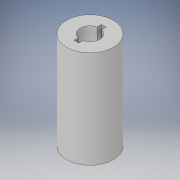
# Autodesk Inventor part: BlenderRoll
Saved by Autodesk Inventor 2019 (Build 230136000, 136)
## iProperties
Created: 2018-06-05
Part Number: BlenderRoll
Material: Ogólny
Document SubType Name: Modeling
Designer: Kamil
Density: 1 g/cm^3
Appearance: Domyślna
Author: Kamil
Autodesk Inventor part; units mm, degrees
ref_plane "YZ Plane" through (0, 0, 0) normal (1, 0, 0) x (0, 1, 0)
ref_plane "XZ Plane" through (0, 0, 0) normal (0, 1, 0) x (-1, 0, 0)
ref_plane "XY Plane" through (0, 0, 0) normal (0, 0, 1) x (1, 0, 0)
sketch "Szkic1" plane through (0, 0, 0) normal (0, 1, 0) x (-1, 0, 0)
  circle A0 centre (2.6768, 3.8124) radius 6
  circle A1 centre (2.6768, 3.8124) radius 2.25
  point P0 (0, 0)
  dimension "d1" = 12
  dimension "d2" = 4.5
  constraints: 2 centre point, 1 coincident
  measures "d1" diameter of A0
  measures "d2" diameter of A1
extrude "Wyciągnięcie proste1" add sketch "Szkic1" along normal blind 12
sketch "Szkic2" plane through (-2.6768, 12, 3.8124) normal (0, 1, 0) x (1, 0, 0)
  point P0 (2.6768, 3.8124)
sketch "Szkic3" plane through (-2.6768, 12, 3.8124) normal (0, 1, 0) x (1, 0, 0)
  point P0 (2.6768, 3.8124)
sketch "Szkic4" plane through (-2.6768, 12, 3.8124) normal (0, 1, 0) x (1, 0, 0)
  circle A0 centre (0, 0) radius 6
  point P0 (2.6768, 3.8124)
  dimension "d5" = 12
  constraints: 1 centre point
  measures "d5" diameter of A0
extrude "Wyciągnięcie proste2" add sketch "Szkic4" along normal blind 5
sketch "Szkic5" plane through (-2.6768, 17, 3.8124) normal (0, 1, 0) x (1, 0, 0)
  circle A0 centre (0, 0) radius 6
  arc A1 (-0.6, 2.4269) -> (-0.6, -2.4269) centre (0, 0) ccw
  line L0 (-0.6, 3.5) -> (0.6, 3.5)
  line L1 (0.6, 3.5) -> (0.6, 2.4269)
  line L2 (-0.6, -3.5) -> (0.6, -3.5)
  line L3 (0.6, -3.5) -> (0.6, -2.4269)
  line L4 (-0.6, 2.4269) -> (-0.6, 3.5)
  arc A2 (0.6, -2.4269) -> (0.6, 2.4269) centre (0, 0) ccw
  line L5 (-0.6, -2.4269) -> (-0.6, -3.5)
  dimension "d8" = 12
  dimension "d10" = 1.2
  dimension "d12" = 1.2
  constraints: 12 end point, 5 point on circle, 3 centre point, 2 parallel, 1 coincident
  measures "d8" diameter of A0
  measures "d10" distance of L0.start L0.end
  measures "d12" distance of L2.end L2.start
extrude "Wyciągnięcie proste3" add sketch "Szkic5" along normal blind 8
